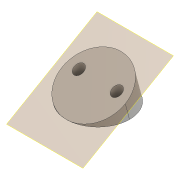
# Autodesk Inventor part: holder_d435_30deg
Saved by Autodesk Inventor 2018 (Build 220112000, 112)
## iProperties
Created: 2018-03-14
Part Number: holder_d435_30deg
Material: Generic
Document SubType Name: Modeling
Designer: Bardo91
Density: 1 g/cm^3
Appearance: Default
Author: Bardo91
Autodesk Inventor part; units mm, degrees
ref_plane "YZ Plane" through (0, 0, 0) normal (1, 0, 0) x (0, 1, 0)
ref_plane "XZ Plane" through (0, 0, 0) normal (0, 1, 0) x (-1, 0, 0)
sketch "Sketch1" plane through (0, 0, 0) normal (0, 0, 1) x (1, 0, 0)
  line L0 (0, 0) -> (0, 10)
  circle A0 centre (0, 10) radius 10
  dimension "d0" = 10
  dimension "d1" = 20
  constraints: 2 end point, 1 centre point, 1 coincident, 1 vertical
  measures "d0" distance of L0.start L0.end
  measures "d1" diameter of A0
ref_plane "Work Plane1" through (0, 0, 0) normal (0, -0.5, 0.866) x (1, 0, 0)
sketch "Sketch2" plane through (0, 0, 0) normal (0, -0.5, 0.866) x (1, 0, 0)
  line L0 (0, 0) -> (0, 10)
  circle A0 centre (0, 10) radius 10
  dimension "d3" = 10
  dimension "d4" = 20
  constraints: 2 end point, 1 centre point, 1 coincident, 1 vertical
  measures "d3" distance of L0.start L0.end
  measures "d4" diameter of A0
loft "Loft1" add profiles "Sketch1", "Sketch2"
sketch "Sketch3" plane through (0, 10, 0) normal (0, 0, -1) x (-1, 0, 0)
  line L0 (0, 0) -> (-6, 0)
  line L1 (0, 0) -> (6, 0)
  circle A0 centre (-6, 0) radius 1.5
  circle A1 centre (6, 0) radius 1.5
  point P0 (0, -10)
  dimension "d9" = 6
  dimension "d10" = 6
  dimension "d11" = 3
  dimension "d12" = 3
  constraints: 4 end point, 2 centre point, 2 coincident, 2 horizontal
  measures "d9" distance of L0.start L0.end
  measures "d10" distance of L0.start L1.end
  measures "d11" diameter of A0
  measures "d12" diameter of A1
extrude "Extrusion1" cut sketch "Sketch3" against normal through all
body "Solid1"
